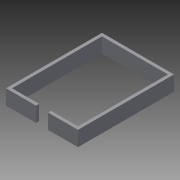
# Autodesk Inventor part: square loop
Saved by Autodesk Inventor 2015 (Build 190159000, 159)
## iProperties
Created: 2014-05-21
Part Number: square loop
Material: Generic
Document SubType Name: Modeling
Designer: jad211
Density: 1 g/cm^3
Appearance: Default
Author: jad211
Autodesk Inventor part; units mm, degrees
ref_plane "YZ Plane" through (0, 0, 0) normal (1, 0, 0) x (0, 1, 0)
ref_plane "XZ Plane" through (0, 0, 0) normal (0, 1, 0) x (-1, 0, 0)
ref_plane "XY Plane" through (0, 0, 0) normal (0, 0, 1) x (1, 0, 0)
sketch "Sketch1" plane through (0, 0, 0) normal (0, 1, 0) x (-1, 0, 0)
  line L0 (-12, 16) -> (12, 16)
  line L1 (12, 16) -> (12, -16)
  line L2 (12, -16) -> (-12, -16)
  line L3 (-12, -16) -> (-12, 16)
  line L4 (11, 15) -> (-11, 15)
  line L5 (-11, 15) -> (-11, -15)
  line L6 (-11, -15) -> (11, -15)
  line L7 (11, -15) -> (11, 15)
  point P0 (0, 0)
  dimension "d0" = 12
  dimension "d1" = 16
  dimension "d2" = 12
  dimension "d3" = 16
  dimension "d4" = 1
  dimension "d5" = 1
  dimension "d6" = 1
  dimension "d7" = 1
  constraints: 16 end point
  measures "d0" distance from line of point (0, 0) L1
  measures "d1" distance from line of point (0, 0) L2
  measures "d2" distance from line of L3 point (0, 0)
  measures "d3" distance from line of point (0, 0) L0
  measures "d4" distance between parallel lines of L0 L4
  measures "d5" distance between parallel lines of L2 L6
  measures "d6" distance between parallel lines of L1 L7
  measures "d7" distance between parallel lines of L3 L5
extrude "Extrusion1" add sketch "Sketch1" along normal blind 5
sketch "Sketch2" plane through (-12, 0, 16) normal (0, 0, 1) x (1, 0, 0)
  line L0 (1, 5) -> (23, 5) projected
  line L1 (23, 0) -> (1, 0) projected
  line L2 (10, 5) -> (14, 5)
  line L3 (14, 5) -> (14, 0)
  line L4 (14, 0) -> (10, 0)
  line L5 (10, 0) -> (10, 5)
  point P0 (12, 0)
  dimension "d10" = 2
  dimension "d11" = 2
  constraints: 8 end point, 2 point on line
  measures "d10" distance from line of point (12, 0) L5
  measures "d11" distance from line of point (12, 0) L3
extrude "Extrusion2" cut sketch "Sketch2" against normal blind 5
equation "\"d2\" = d0"
equation "\"d3\" = d1"
equation "\"d5\" = d4"
equation "\"d6\" = d4"
equation "\"d7\" = d4"
equation "\"d11\" = d10"
body "Solid1"
